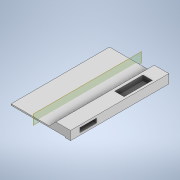
# Autodesk Inventor part: Mock Acer SB230
Saved by Autodesk Inventor 2022 (Build 260153000, 153)
## iProperties
Created: 2021-07-16
Part Number: Mock Acer SB230
Material: Generic
Document SubType Name: Modeling
Designer: negre
Density: 1 g/cm^3
Appearance: Default
Author: negre
Comments: Take care to not block the ports on the back or the buttons on the bottom.
Autodesk Inventor part; units mm, degrees
ref_plane "YZ Plane" through (0, 0, 0) normal (1, 0, 0) x (0, 1, 0)
ref_plane "XZ Plane" through (0, 0, 0) normal (0, 1, 0) x (-1, 0, 0)
ref_plane "XY Plane" through (0, 0, 0) normal (0, 0, 1) x (1, 0, 0)
sketch "Sketch1" plane through (0, 0, 0) normal (0, 1, 0) x (-1, 0, 0)
  line L0 (-40.1461, 220.4385) -> (-360.1461, 220.4385)
  line L1 (-360.1461, 220.4385) -> (-360.1461, -309.5615)
  line L2 (-360.1461, -309.5615) -> (-40.1461, -309.5615)
  line L3 (-40.1461, -309.5615) -> (-40.1461, 220.4385)
  point P0 (0, 0)
  dimension "d0" = 530
  dimension "d1" = 320
  constraints: 8 end point, 2 parallel, 1 horizontal, 1 perpendicular
  measures "d0" distance between parallel lines of L2 L0
  measures "d1" distance between parallel lines of L1 L3
extrude "Extrusion1" add sketch "Sketch1" along normal blind 7
sketch "Sketch7" plane through (0, 0, 0) normal (0, -1, 0) x (1, 0, 0)
  line L0 (360.1461, 220.4385) -> (360.1461, -309.5615) projected
  line L1 (40.1461, 220.4385) -> (360.1461, 220.4385) projected
  line L2 (360.1461, -309.5615) -> (331.5711, -309.5615)
  line L3 (331.5711, -309.5615) -> (331.5711, 220.4385)
  line L4 (331.5711, 220.4385) -> (360.1461, 220.4385)
  line L5 (360.1461, 220.4385) -> (360.1461, -309.5615)
  point P0 (0, 0)
  dimension "d15" = 28.575
  constraints: 8 end point, 2 parallel, 1 horizontal, 1 perpendicular, 1 point on line
  measures "d15" distance of L0.end L2.end
extrude "Extrusion5" add sketch "Sketch7" along normal blind 5.08
sketch "Sketch8" plane through (0, 7, 0) normal (0, 1, 0) x (1, 0, 0)
  line L0 (360.1461, -220.4385) -> (360.1461, 309.5615) projected
  line L1 (360.1461, 309.5615) -> (40.1461, 309.5615) projected
  line L2 (360.1461, -220.4385) -> (283.9461, -220.4385)
  line L3 (283.9461, -220.4385) -> (283.9461, 309.5615)
  line L4 (283.9461, 309.5615) -> (360.1461, 309.5615)
  line L5 (360.1461, 309.5615) -> (360.1461, -220.4385)
  point P0 (0, 0)
  dimension "d18" = 76.2
  constraints: 8 end point, 2 parallel, 1 horizontal, 1 perpendicular, 1 point on line
  measures "d18" distance of L0.start L2.end
extrude "Extrusion6" add sketch "Sketch8" along normal blind 36.068
sketch "Sketch9" plane through (0, 7, 0) normal (0, 1, 0) x (1, 0, 0)
  line L0 (283.9461, 309.5615) -> (283.9461, -220.4385) projected
  line L1 (283.9461, 309.5615) -> (40.1461, 309.5615) projected
  line L2 (283.9461, -220.4385) -> (245.8461, -220.4385)
  line L3 (245.8461, -220.4385) -> (245.8461, 309.5615)
  line L4 (245.8461, 309.5615) -> (283.9461, 309.5615)
  line L5 (283.9461, 309.5615) -> (283.9461, -220.4385)
  point P0 (0, 0)
  dimension "d21" = 38.1
  constraints: 8 end point, 2 parallel, 1 horizontal, 1 perpendicular, 1 point on line
  measures "d21" distance of L0.end L2.end
extrude "Extrusion7" add sketch "Sketch9" along normal blind 36.068
chamfer "Chamfer1" distance 35.56 angle 45 1 edges at (245.8461, 43.068, -44.5615) measured on face at (245.8461, 19.0227, -132.8949)
sketch "Sketch10" plane through (0, 43.068, 0) normal (0, 1, 0) x (1, 0, 0)
  line L0 (296.6461, 80.9615) -> (347.4461, 80.9615)
  line L1 (347.4461, 80.9615) -> (347.4461, 233.3615)
  line L2 (347.4461, 233.3615) -> (296.6461, 233.3615)
  line L3 (296.6461, 233.3615) -> (296.6461, 80.9615)
  line L4 (360.1461, 309.5615) -> (281.4061, 309.5615) projected
  line L5 (360.1461, -220.4385) -> (360.1461, 309.5615) projected
  point P0 (0, 0)
  dimension "d27" = 76.2
  dimension "d28" = 228.6
  dimension "d29" = 12.7
  dimension "d30" = 63.5
  constraints: 8 end point, 2 parallel, 1 horizontal, 1 perpendicular
  measures "d27" distance between parallel lines of L4 L2
  measures "d28" distance between parallel lines of L4 L0
  measures "d29" distance between parallel lines of L5 L1
  measures "d30" distance between parallel lines of L5 L3
extrude "Extrusion8" cut sketch "Sketch10" against normal blind 25.4
sketch "Sketch11" plane through (360.1461, -5.08, 220.4385) normal (1, 0, 0) x (0, 0, -1)
  line L0 (530, 12.588) -> (0, 12.588) projected
  line L1 (50.8, 35.56) -> (139.7, 35.56)
  line L2 (139.7, 35.56) -> (139.7, 12.588)
  line L3 (139.7, 12.588) -> (50.8, 12.588)
  line L4 (50.8, 12.588) -> (50.8, 35.56)
  line L5 (0, 48.148) -> (0, 0) projected
  line L6 (530, 0) -> (0, 0) projected
  line L7 (0, 48.148) -> (530, 48.148) projected
  point P0 (220.4385, 5.08)
  dimension "d33" = 50.8
  dimension "d34" = 139.7
  dimension "d35" = 12.588
  dimension "d36" = 12.588
  constraints: 8 end point, 2 parallel, 1 horizontal, 1 perpendicular, 1 point on line
  measures "d33" distance between parallel lines of L5 L4
  measures "d34" distance between parallel lines of L5 L2
  measures "d35" distance between parallel lines of L6 L0
  measures "d36" distance between parallel lines of L7 L1
extrude "Extrusion9" cut sketch "Sketch11" against normal blind 25.4
ref_plane "Work Plane2" through (185.8586, 0, -309.5615) normal (-1, 0, 0) x (0, 0, 1)
equation "\"d36\" = d35"
body "Solid1"
